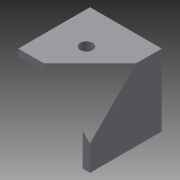
# Autodesk Inventor part: dociskacz
Saved by Autodesk Inventor 2015 (Build 190159000, 159)
## iProperties
Created: 2015-05-04
Part Number: dociskacz
Material: Ogólny
Document SubType Name: Modeling
Designer: Kuba
Density: 1 g/cm^3
Appearance: Domyślna
Author: Kuba
Autodesk Inventor part; units mm, degrees
ref_plane "YZ Plane" through (0, 0, 0) normal (1, 0, 0) x (0, 1, 0)
ref_plane "XZ Plane" through (0, 0, 0) normal (0, 1, 0) x (-1, 0, 0)
ref_plane "XY Plane" through (0, 0, 0) normal (0, 0, 1) x (1, 0, 0)
sketch "Szkic1" plane through (0, 0, 0) normal (0, 1, 0) x (-1, 0, 0)
  line L0 (0, 0) -> (20, 0)
  line L1 (0, -20) -> (0, 0)
  line L2 (20, 0) -> (20, -2)
  line L3 (20, -2) -> (2, -2)
  line L4 (2, -2) -> (2, -20)
  line L5 (2, -20) -> (0, -20)
  dimension "d2" = 2
  dimension "d3" = 18
  dimension "d4" = 20
  dimension "d5" = 18
  dimension "d6" = 2
  constraints: 12 end point, 3 perpendicular, 2 horizontal
  measures "d2" distance of L0.end L2.end
  measures "d3" distance of L2.end L3.end
  measures "d4" distance of L1.start L0.start
  measures "d5" distance of L3.end L4.end
  measures "d6" distance of L4.end L1.start
extrude "Wyciągnięcie proste1" add sketch "Szkic1" along normal blind 20
sketch "Szkic2" plane through (-2, 0, -2) normal (0, 0, -1) x (-1, 0, 0)
  line L0 (18, 0) -> (0, 0) projected
  line L1 (18, 0) -> (18, 20) projected
  line L2 (0, 20) -> (18, 20) projected
  line L3 (0, 0) -> (0, 20) projected
  point P0 (-2, 0)
  point P1 (9, 10)
  dimension "d9" = 10
  dimension "d10" = 10
  dimension "d11" = 9
  dimension "d12" = 9
  measures "d9" distance from line of L2 point (9, 10)
  measures "d10" distance from line of L0 point (9, 10)
  measures "d11" distance from line of L1 point (9, 10)
  measures "d12" distance from line of L3 point (9, 10)
hole "Otwór1" at (-11, 10, -2) direction (0, 0, 1) diameter 3.5 end through all
equation "\"d9\" = d10"
equation "\"d11\" = d12"
